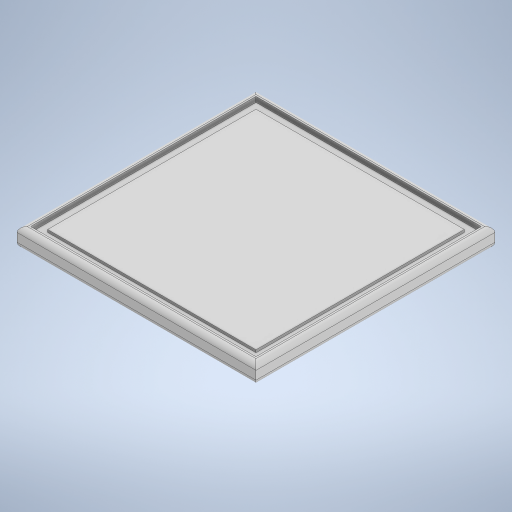
# Autodesk Inventor part: OV-PAM_n_4_bottom
Saved by Autodesk Inventor 2024 (Build 280153000, 153)
## iProperties
Created: 2023-08-31
Part Number: OV-PAM_n_4_bottom
Material: 일반
Document SubType Name: Modeling
Designer: jsw
Density: 1 g/cm^3
Appearance: 기본값
Author: jsw
Autodesk Inventor part; units mm, degrees
ref_plane "YZ Plane" through (0, 0, 0) normal (1, 0, 0) x (0, 1, 0)
ref_plane "XZ Plane" through (0, 0, 0) normal (0, 1, 0) x (-1, 0, 0)
ref_plane "XY Plane" through (0, 0, 0) normal (0, 0, 1) x (1, 0, 0)
sketch "스케치1" plane through (0, 0, 0) normal (0, 1, 0) x (-1, 0, 0)
  line L0 (-24.9446, -24.9446) -> (24.9446, -24.9446)
  line L1 (24.9446, -24.9446) -> (24.9446, 24.9446)
  line L2 (24.9446, 24.9446) -> (-24.9446, 24.9446)
  line L3 (-24.9446, 24.9446) -> (-24.9446, -24.9446)
  line L4 (-24.9446, -24.9446) -> (24.9446, 24.9446) construction
  line L5 (24.9446, -24.9446) -> (-24.9446, 24.9446) construction
  line L6 (-28.1446, -28.1446) -> (28.1446, -28.1446)
  line L7 (28.1446, -28.1446) -> (28.1446, 28.1446)
  line L8 (28.1446, 28.1446) -> (-28.1446, 28.1446)
  line L9 (-28.1446, 28.1446) -> (-28.1446, -28.1446)
  line L10 (-28.1446, -28.1446) -> (28.1446, 28.1446) construction
  line L11 (28.1446, -28.1446) -> (-28.1446, 28.1446) construction
  point P0 (0, 0)
  dimension "d0" = 70.554
  dimension "d1" = 3.2
  constraints: 24 end point, 4 midpoint, 4 parallel, 4 perpendicular, 2 horizontal
  measures "d0" distance of L2.end L0.end
  measures "d1" distance between parallel lines of L1 L7
extrude "돌출1" add sketch "스케치1" along normal blind 4.4 contours L3 L2 L1 L0 | L9 L8 L7 L6
sketch "스케치2" plane through (0, 4.4, 0) normal (0, 1, 0) x (1, 0, 0)
  line L0 (-28.1446, 28.1446) -> (-28.1446, -28.1446) projected
  line L1 (-28.1446, -28.1446) -> (28.1446, -28.1446) projected
  line L2 (28.1446, -28.1446) -> (28.1446, 28.1446) projected
  line L3 (28.1446, 28.1446) -> (-28.1446, 28.1446) projected
  line L4 (26.5446, 26.5446) -> (-26.5446, 26.5446)
  line L5 (-26.5446, 26.5446) -> (-26.5446, -26.5446)
  line L6 (-26.5446, -26.5446) -> (26.5446, -26.5446)
  line L7 (26.5446, -26.5446) -> (26.5446, 26.5446)
  line L8 (26.5446, 26.5446) -> (-26.5446, -26.5446) construction
  line L9 (-26.5446, 26.5446) -> (26.5446, -26.5446) construction
  line L10 (24.5446, 24.5446) -> (-24.5446, 24.5446)
  line L11 (-24.5446, 24.5446) -> (-24.5446, -24.5446)
  line L12 (-24.5446, -24.5446) -> (24.5446, -24.5446)
  line L13 (24.5446, -24.5446) -> (24.5446, 24.5446)
  line L14 (24.5446, 24.5446) -> (-24.5446, -24.5446) construction
  line L15 (-24.5446, 24.5446) -> (24.5446, -24.5446) construction
  point P0 (0, 0)
  point P1 (0, 28.1446)
  point P2 (-28.1446, 0)
  dimension "d4" = 1.6
  dimension "d5" = 2
  constraints: 24 end point, 6 midpoint, 4 parallel, 3 perpendicular, 2 horizontal, 1 horizontal alignment, 1 point on line, 1 vertical alignment
  measures "d4" distance between parallel lines of L5 L0
  measures "d5" distance between parallel lines of L11 L5
extrude "돌출2" cut sketch "스케치2" against normal blind 1.2 contours L7 L6 L5 L4 | L13 L12 L11 L10
sketch "스케치3" plane through (0, 3.2, 0) normal (0, 1, 0) x (1, 0, 0)
  line L0 (24.5446, 24.5446) -> (-24.5446, 24.5446)
  line L1 (-24.5446, 24.5446) -> (-24.5446, -24.5446)
  line L2 (-24.5446, -24.5446) -> (24.5446, -24.5446)
  line L3 (24.5446, -24.5446) -> (24.5446, 24.5446)
  line L4 (24.5446, 24.5446) -> (-24.5446, -24.5446) construction
  line L5 (-24.5446, 24.5446) -> (24.5446, -24.5446) construction
  line L6 (-26.5446, -26.5446) -> (-26.5446, 26.5446) projected
  point P0 (0, 0)
  dimension "d8" = 2
  constraints: 12 end point, 2 midpoint, 2 parallel, 2 perpendicular, 1 horizontal
  measures "d8" distance between parallel lines of L1 L6
extrude "돌출3" add sketch "스케치3" along normal blind 0.6
fillet "모깎기1" radius 1.2 8 edges at (0, 4.4, 28.1446) (28.1446, 4.4, 0) (0, 4.4, -28.1446) (-28.1446, 4.4, 0) (-28.1446, 0, 0) (0, 0, 28.1446) (28.1446, 0, 0) (0, 0, -28.1446)
sketch "스케치6" plane through (0, 0, 0) normal (0, -1, 0) x (1, 0, 0)
  circle A0 centre (0, 0) radius 3.9687
  dimension "d27" = 7.9375
  constraints: 1 centre point, 1 coincident
  measures "d27" diameter of A0
extrude "돌출6" add sketch "스케치6" along normal blind 7.62
thread "스레드1" size "5/16-18 UNC" class "2A" standard "ANSI Unified Screw Threads" full length
